Cyclone  Cyclone to Saw Hose Adapter (Autodesk Fusion 360 design; units mm, degrees)
Autodesk Fusion 360 part; units mm, degrees
sketch "Sketch1" plane through (0, 0, 0) normal (0, 0, 1) x (1, 0, 0)
  circle A0 centre (0, 0) radius 22.75
  circle A1 centre (0, 0) radius 24.25
  dimension "d1" = 45.5
  dimension "d2" = 48.5
  constraint coincident A0.centre A1.centre
  measures "d1" diameter of A0
  measures "d2" diameter of A1
extrude "Extrude1" add sketch "Sketch1" along normal blind 33
sketch "Sketch2" plane through (0, 0, 0) normal (0, 1, 0) x (1, 0, 0)
  line L0 (-24.25, 0) -> (24.25, 0)
  line L1 (4.75, -6.25) -> (-4.75, -6.25)
  line L2 (-4.75, -6.25) -> (-4.75, -2.75)
  line L3 (-4.75, -2.75) -> (4.75, -2.75)
  line L4 (4.75, -2.75) -> (4.75, -6.25)
  line L5 (4.75, -6.25) -> (-4.75, -2.75) construction
  line L6 (-4.75, -6.25) -> (4.75, -2.75) construction
  point P0 (0, -4.5)
  dimension "d9" = 9.5
  dimension "d10" = 3.5
  dimension "d11" = 2.75
  constraint perpendicular L1 L2
  constraint parallel L1 L3
  constraint parallel L2 L4
  constraint horizontal L1
  constraint coincident L5 P0
  constraint coincident L6 P0
  constraint vertical origin P0
  measures "d9" distance of L2.end L3.end
  measures "d10" distance of L1.end L2.end
  measures "d11" distance of origin L3
extrude "Extrude2" cut sketch "Sketch2" along normal mid plane 66
sketch "Sketch3" plane through (0, 0, 33) normal (0, 0, 1) x (-1, 0, 0)
  circle A0 centre (0, 0) radius 22.75
  circle A1 centre (0, 0) radius 24.25
  circle A2 centre (0, 0) radius 25
  circle A3 centre (0, 0) radius 22.75
  constraint concentric A0 A2
  constraint concentric A2 A3
  measures "d14" diameter of A2
  measures "d15" diameter of A3
extrude "Extrude3" add sketch "Sketch3" along normal blind 3 contours A1 | A2
sketch "Sketch4" plane through (0, 0, 36) normal (0, 0, 1) x (-1, 0, 0)
  circle A0 centre (0, 0) radius 22.75
  circle A1 centre (0, 0) radius 25
  circle A2 centre (0, 0) radius 23.25
  circle A3 centre (0, 0) radius 22
  dimension "d18" = 46.5
  dimension "d19" = 44
  constraint coincident A0.centre A1.centre
  measures "d18" diameter of A2
  measures "d19" diameter of A3
ref_plane "WorkPlane2" through (0, 0, 43) normal (0, 0, 1) x (-1, 0, 0)
sketch "Sketch6" plane through (0, 0, 43) normal (0, 0, 1) x (1, 0, 0)
  circle A0 centre (0, 0) radius 22
  circle A1 centre (0, 0) radius 23.25
  dimension "d26" = 44
  dimension "d27" = 46.5
  constraint coincident A0.centre A1.centre
  measures "d26" diameter of A0
  measures "d27" diameter of A1
extrude "Extrude4" add sketch "Sketch6" against normal blind 7
ref_plane "WorkPlane1" through (0, 0, 56) normal (0, 0, 1) x (-1, 0, 0)
sketch "Sketch5" plane through (0, 0, 56) normal (0, 0, 1) x (1, 0, 0)
  circle A0 centre (0, 0) radius 22.75
  circle A1 centre (0, 0) radius 21.25
  dimension "d21" = 45.5
  dimension "d22" = 42.5
  constraint coincident A0.centre A1.centre
  measures "d21" diameter of A0
  measures "d22" diameter of A1
loft "Loft1" add profiles "Sketch6", "Sketch5" section 1 section 2
loft "Loft2" cut profiles "Sketch5", "Sketch6" section 1 contours A1 section 2 contours A0
chamfer "Chamfer1" distance 1.75 angle 45 1 edges at (-21.6766, 8.4076, 36)
chamfer "Chamfer3" distance 0.75 angle 45 1 edges at (21.2104, -8.2268, 36)
chamfer "Chamfer4" distance 0.75 angle 45 1 edges at (-22.6089, -8.7692, 33)
fillet "Fillet1" radius 1.75 8 edges at (-4.75, -23.0144, 6.25) (-4.75, -23.0144, 2.75) (4.75, -23.0144, 6.25) (4.75, -23.0144, 2.75) (4.75, 23.0144, 2.75) (4.75, 23.0144, 6.25) (-4.75, 23.0144, 6.25) (-4.75, 23.0144, 2.75)
